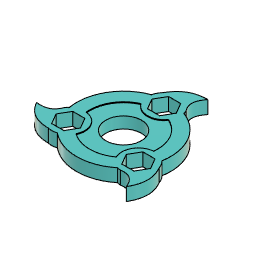
fidgetspinner (Autodesk Fusion 360 design; units mm, degrees)
Autodesk Fusion 360 part; units mm, degrees
sketch "Sketch1" plane through (0, 0, 0) normal (0, 0, 1) x (1, 0, 0) in component "Figet Spinner"
  circle A0 centre (0, 0) radius 25 construction
  line L0 (0, 0) -> (0, 37) construction
  line L1 (-3.7528, 31.5) -> (-7.5056, 25)
  line L2 (-7.5056, 25) -> (-3.7528, 18.5)
  line L3 (-3.7528, 18.5) -> (3.7528, 18.5)
  line L4 (3.7528, 18.5) -> (7.5056, 25)
  line L5 (7.5056, 25) -> (3.7528, 31.5)
  line L6 (3.7528, 31.5) -> (-3.7528, 31.5)
  spline S0 degree 5 poles (-7.5138, 31.9717) (-7.2318, 32.4496) (-6.6528, 33.3792) (-5.7393, 34.6951) (-4.4298, 36.2901) (-2.6362, 38.0009) (-0.6893, 39.4059) (1.3878, 40.4856) (3.5405, 41.2348) (5.6614, 41.6834) (7.5834, 41.9073) (8.8194, 41.9749) (9.5098, 41.9954) (9.8557, 42) (10, 42) knots 0 0 0 0 0 0 0.1 0.2 0.3 0.4 0.5 0.6 0.7 0.8 0.9 1 1 1 1 1 1
  line L7 (9, 42) -> (11, 42)
  spline S1 degree 5 poles (10, 42) (9.5694, 41.4679) (8.784, 40.4086) (7.8329, 38.8347) (7.0266, 36.7666) (6.8325, 34.2352) (7.3693, 32.2479) (8.175, 30.7821) (8.8868, 29.8139) (9.2884, 29.3289) (9.2944, 29.3216) knots 0 0 0 0 0 0 0.1 0.2 0.3 0.4 0.5 0.501529 0.501529 0.501529 0.501529 0.501529 0.501529
  line L8 (8.3624, 30.4454) -> (10.2264, 28.1979)
  circle A1 centre (0, 0) radius 11
  spline S2 degree 5 poles (-23.9314, -22.493) (-24.4863, -22.4877) (-25.5808, -22.451) (-27.1772, -22.3179) (-29.2133, -21.9813) (-31.5916, -21.2835) (-33.7818, -20.2999) (-35.7555, -19.0409) (-37.4806, -17.5512) (-38.9296, -15.9388) (-40.0844, -14.3862) (-40.7611, -13.3496) (-41.124, -12.762) (-41.3009, -12.4647) (-41.3731, -12.3397) knots 0 0 0 0 0 0 0.1 0.2 0.3 0.4 0.5 0.6 0.7 0.8 0.9 1 1 1 1 1 1
  spline S3 degree 5 poles (-41.3731, -12.3397) (-40.6969, -12.4466) (-39.3869, -12.5972) (-37.5483, -12.6339) (-35.3541, -12.2981) (-33.0648, -11.2004) (-31.6122, -9.742) (-30.7456, -8.3113) (-30.263, -7.2107) (-30.0438, -6.6205) (-30.0405, -6.6116) knots 0 0 0 0 0 0 0.1 0.2 0.3 0.4 0.5 0.501529 0.501529 0.501529 0.501529 0.501529 0.501529
  line L9 (-25.4034, -6) -> (-29.1562, -12.5)
  line L10 (-29.1562, -12.5) -> (-25.4034, -19)
  line L11 (-25.4034, -19) -> (-17.8979, -19)
  line L12 (-17.8979, -19) -> (-14.1451, -12.5)
  line L13 (-14.1451, -12.5) -> (-17.8979, -6)
  line L14 (-17.8979, -6) -> (-25.4034, -6)
  spline S4 degree 5 poles (31.4452, -9.4787) (31.7181, -9.9619) (32.2336, -10.9281) (32.9164, -12.3772) (33.643, -14.3087) (34.2278, -16.7174) (34.4712, -19.106) (34.3677, -21.4447) (33.9401, -23.6836) (33.2682, -25.7446) (32.5011, -27.521) (31.9416, -28.6253) (31.6142, -29.2335) (31.4452, -29.5353) (31.3731, -29.6603) knots 0 0 0 0 0 0 0.1 0.2 0.3 0.4 0.5 0.6 0.7 0.8 0.9 1 1 1 1 1 1
  spline S5 degree 5 poles (31.3731, -29.6603) (31.1275, -29.0213) (30.6029, -27.8115) (29.7154, -26.2009) (28.3275, -24.4685) (26.2323, -23.0347) (24.2429, -22.506) (22.5706, -22.4708) (21.3762, -22.6032) (20.7554, -22.7084) (20.7461, -22.71) knots 0 0 0 0 0 0 0.1 0.2 0.3 0.4 0.5 0.501529 0.501529 0.501529 0.501529 0.501529 0.501529
  line L15 (17.8979, -19) -> (25.4034, -19)
  line L16 (25.4034, -19) -> (29.1562, -12.5)
  line L17 (29.1562, -12.5) -> (25.4034, -6)
  line L18 (25.4034, -6) -> (17.8979, -6)
  line L19 (17.8979, -6) -> (14.1451, -12.5)
  line L20 (14.1451, -12.5) -> (17.8979, -19)
  arc A2 (-8.464, 19.2188) -> (-20.8759, -2.2793) centre (0, 0) ccw
  arc A3 (-12.4119, -16.9394) -> (12.4119, -16.9394) centre (0, 0) ccw
  arc A4 (20.8759, -2.2793) -> (8.464, 19.2188) centre (0, 0) ccw
  arc A5 (-18.5686, -22.2757) -> (18.5686, -22.2757) centre (0, 0) ccw
  arc A6 (28.5756, -4.9431) -> (10.007, 27.2188) centre (0, 0) ccw
  arc A7 (-8.464, 19.2188) -> (8.464, 19.2188) centre (0, 25) ccw
  arc A8 (-7.5138, 31.9717) -> (-10.007, 27.2187) centre (0, 25) ccw
  arc A9 (18.5686, -22.2757) -> (20.7461, -22.71) centre (21.6506, -12.5) ccw
  arc A10 (31.4452, -9.4787) -> (28.5756, -4.9431) centre (21.6506, -12.5) ccw
  arc A11 (20.8759, -2.2793) -> (12.4119, -16.9394) centre (21.6506, -12.5) ccw
  arc A12 (-10.007, 27.2187) -> (-28.5756, -4.9431) centre (0, 0) ccw
  arc A13 (-28.5756, -4.9431) -> (-30.0405, -6.6116) centre (-21.6506, -12.5) ccw
  arc A14 (-23.9314, -22.493) -> (-18.5686, -22.2757) centre (-21.6506, -12.5) ccw
  arc A15 (-12.4119, -16.9394) -> (-20.8759, -2.2793) centre (-21.6506, -12.5) ccw
  arc A16 (10.007, 27.2187) -> (9.2944, 29.3217) centre (0, 25) ccw
  arc A17 (7.7553, 31.702) -> (7.7553, 31.702) centre (0, 25) ccw
  point P0 (0, 25)
  point P1 (3, 41)
  point P2 (-37.007, -17.9019)
  point P3 (-31.3324, -9.1347)
  point P4 (34.007, -23.0981)
  point P5 (23.5771, -22.5673)
  dimension "d14" = 50
  dimension "d15" = 6.5
  dimension "d16" = 31.5
  dimension "d17" = 20.5
  dimension "d18" = 22
  constraint coincident A0.centre L0.start
  constraint vertical L0
  constraint coincident A0 P0
  constraint coincident L0 P0
  constraint coincident P0 A7.centre
  constraint coincident S0.start A7
  constraint midpoint S0.end L7
  constraint coincident A17.start A7
  constraint coincident S1.end A7
  constraint midpoint S1.end L8
  constraint concentric A0 A3
  constraint coincident A3.start A14
  constraint concentric A0 A5
  constraint coincident A12.end A14
  constraint concentric A2 A3
  constraint coincident A4.start A10
  constraint concentric A3 A4
  constraint concentric A5 A6
  constraint concentric A7 A16
  constraint coincident S1 A17.start
  constraint concentric A8 A16
  constraint coincident A5.end A10
  constraint concentric A9 A10
  constraint concentric A10 A11
  constraint concentric A13 A14
  constraint concentric A14 A15
  constraint coincident S1 A16.end
  constraint concentric A16 A17
  constraint coincident S5 A9.end
  constraint coincident S3 A13.end
  measures "d14" diameter of A0
  measures "d15" distance of P0 L6
  measures "d16" distance of A0.centre L6
  measures "d17" diameter of A7
  measures "d18" diameter of A1
extrude "Extrude2" add sketch "Sketch1" along normal mid plane 8 contours S1 A7 A8 A16 A17 | S0 S1 A17 | S2 S3 S4 S5 A2 A3 A4 A5 A6 A9 A10 A11 A12 A13 A14 A15 A17 in component "Figet Spinner"
extrude "Extrude3" add sketch "Sketch1" along normal mid plane 7 contours A2 A3 A4 A7 A11 A15 A17 in component "Figet Spinner"
component "Figet Spinner" placed x (1, 0, 0) y (0, 1, 0) z (0, 0, 1) at (0, 0, 0)
